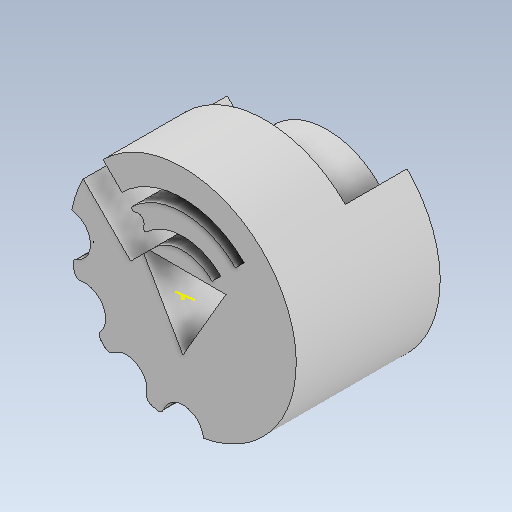
# Autodesk Inventor part: HandleGear
Saved by Autodesk Inventor 2021 (Build 250183000, 183)
## iProperties
Created: 2021-03-14
Part Number: HandleGear
Material: Generic
Document SubType Name: Modeling
Designer: ben
Density: 1 g/cm^3
Appearance: Default
Mass: 73.1754 g
Surface Area: 125.549 cm^2
Volume: 73.1754 cm^3
Author: ben
Autodesk Inventor part; units mm, degrees
ref_plane "YZ Plane" through (0, 0, 0) normal (1, 0, 0) x (0, 1, 0)
ref_plane "XZ Plane" through (0, 0, 0) normal (0, 1, 0) x (-1, 0, 0)
ref_plane "XY Plane" through (0, 0, 0) normal (0, 0, 1) x (1, 0, 0)
sketch "Sketch1" plane through (0, 0, 0) normal (0, 0, 1) x (1, 0, 0)
  line L0 (5.1877, -3.0147) -> (-0.0339, -12) projected
  line L1 (-0.0339, -12) -> (-5.2046, -2.9853) projected
  line L2 (-10.3753, 6.0293) -> (0.0169, 6) projected
  circle A0 centre (0, 0) radius 27.5 projected
  circle A1 centre (0, 0) radius 22.5
  line L3 (0, 27.5) -> (0, 14.4902)
  line L4 (0, 0) -> (27.5, 0) construction
  line L5 (0, 0) -> (27.5, 0) construction
  circle A2 centre (-27.5, 0) radius 5
  circle A3 centre (-23.8157, -13.75) radius 5
  circle A4 centre (-13.75, -23.8157) radius 5
  circle A5 centre (0, -27.5) radius 5
  line L6 (-5.2046, -2.9853) -> (-10.3753, 6.0293) projected
  line L7 (0.0169, 6) -> (10.4092, 5.9706) projected
  line L8 (10.4092, 5.9706) -> (5.1877, -3.0147) projected
  arc A6 (7.0711, 7.0711) -> (-7.0711, 7.0711) centre (0, 0) ccw
  line L9 (0, 0) -> (-7.0711, 7.0711) construction
  line L10 (0, 0) -> (10, 0) construction
  line L11 (0, 0) -> (7.0711, 7.0711) construction
  arc A7 (9.1924, 9.1924) -> (-9.1924, 9.1924) centre (0, 0) ccw
  line L12 (0, 0) -> (-9.1924, 9.1924) construction
  line L13 (0, 0) -> (13, 0) construction
  line L14 (0, 0) -> (9.1924, 9.1924) construction
  arc A8 (12.7279, 12.7279) -> (-12.7279, 12.7279) centre (0, 0) ccw
  line L15 (0, 0) -> (-12.7279, 12.7279) construction
  line L16 (0, 0) -> (18, 0) construction
  line L17 (0, 0) -> (12.7279, 12.7279) construction
  arc A9 (14.8492, 14.8492) -> (-14.8492, 14.8492) centre (0, 0) ccw
  line L18 (0, 0) -> (19, 0) construction
  line L19 (0, 0) -> (14.8492, 14.8492) construction
  line L20 (-7.0711, 7.0711) -> (-9.1924, 9.1924)
  line L21 (-9.1924, 9.1924) -> (-12.7279, 12.7279)
  line L22 (-14.8492, 14.8492) -> (-12.7279, 12.7279)
  line L23 (7.0711, 7.0711) -> (9.1924, 9.1924)
  line L24 (9.1924, 9.1924) -> (12.7279, 12.7279)
  line L25 (14.8492, 14.8492) -> (12.7279, 12.7279)
  line L26 (-7.0711, 7.0711) -> (-9.1924, 9.1924)
  line L27 (-9.1924, 9.1924) -> (-12.7279, 12.7279)
  line L28 (-14.8492, 14.8492) -> (-12.7279, 12.7279)
  line L29 (-7.0711, 7.0711) -> (-19.4454, 19.4454)
  line L30 (-19.4454, 19.4454) -> (-25.1023, 13.7886)
  line L31 (-25.1023, 13.7886) -> (-12.7279, 1.4142)
  line L32 (-12.7279, 1.4142) -> (-7.0711, 7.0711)
  arc A10 (16.9706, 16.9706) -> (-16.9706, 16.9706) centre (0, 0) ccw
  line L33 (-14.8492, 14.8492) -> (-16.9706, 16.9706)
  line L34 (14.8492, 14.8492) -> (16.9706, 16.9706)
  arc A11 (-9.8995, 9.8995) -> (-12.0208, 12.0208) centre (-10.9602, 10.9602) ccw
  point P0 (0, 0)
  point P1 (-27.0822, 4.7753)
  point P2 (4.7753, -27.0822)
  point P3 (-4.9793, -27.0455)
  point P4 (4.9793, -27.0455)
  point P5 (-27.0455, 4.9793)
  point P6 (-27.0455, -4.9793)
  point P7 (-25.9117, -9.2105)
  point P8 (-20.9324, -17.8349)
  point P9 (-17.8349, -20.9324)
  point P10 (-9.2105, -25.9117)
  point P11 (0, -22.5)
  point P12 (-11.25, -19.4856)
  point P13 (-19.4856, -11.25)
  point P14 (-22.5, 0)
  point P15 (-27.0455, 4.9793)
  point P16 (4.9793, -27.0455)
  point P17 (-24.2613, 12.9476)
  dimension "d9" = 10
  dimension "d0" = 5
  dimension "d12" = 90
  dimension "d70" = 10
  dimension "d71" = 135
  dimension "d72" = 90
  dimension "d73" = 13
  dimension "d74" = 135
  dimension "d75" = 90
  dimension "d76" = 18
  dimension "d77" = 135
  dimension "d78" = 90
  dimension "d79" = 21
  dimension "d88" = 8
  dimension "d93" = 24
  dimension "d94" = 3
  constraints: 58 end point, 14 point on circle, 9 centre point, 6 horizontal, 5 coincident, 5 point on line, 3 equal length, 2 parallel, 2 vertical, 1 perpendicular, 21 other
  measures "d70" radius of A6
  measures "d71" angle of L10 L9
  measures "d72" angle of L11 L9
  measures "d73" radius of A7
  measures "d74" angle of L13 L12
  measures "d75" angle of L14 L12
  measures "d76" radius of A8
  measures "d77" angle of L16 L15
  measures "d78" angle of L17 L15
  measures "d79" radius of A9
  measures "d88" distance of L30.end L29.end
  measures "d93" radius of A10
  measures "d94" diameter of A11
extrude "Extrusion6" add sketch "Sketch1" along normal blind 35 contours L8 L7 L2 L32 A6 L23 L24 L25 L34 A1 L31 L6 L1 L0 | A1 A2 A0 L31 | L21 A11 A8 L24 A7 | L29 A10 L3 A1 | A1 L3 A9 L29 | A1 A3 A0 A2 | L3 A10 L34 A1 | A1 L34 A9 L3 | L29 A0 L3 A10 | A1 A4 A0 A3 | L34 A10 L3 A0 A5 A1 | A1 A5 A0 A4
sketch "Sketch7" plane through (0, 0, 0) normal (0, 0, -1) x (-1, 0, 0)
  line L0 (8.6461, 5.0244) -> (4.3372, -2.4878)
  arc A0 (-4.323, -2.5122) -> (4.3372, -2.4878) centre (0, 0) ccw
  line L1 (0.0282, -10) -> (-4.323, -2.5122)
  line L2 (4.3372, -2.4878) -> (0.0282, -10)
  arc A1 (4.3372, -2.4878) -> (-0.0141, 5) centre (0, 0) ccw
  line L3 (-0.0141, 5) -> (8.6461, 5.0244)
  arc A2 (-0.0141, 5) -> (-4.323, -2.5122) centre (0, 0) ccw
  line L4 (-4.323, -2.5122) -> (-8.6743, 4.9755)
  line L5 (-8.6743, 4.9755) -> (-0.0141, 5)
  circle A3 centre (0, 0) radius 27.5
  spline S0 degree 2 poles (19.7349, 0.4642) (19.3981, 0.44) (19.187, 0.6034) knots 0 0 0 1 1 1
  spline S1 degree 2 poles (19.187, 0.6034) (18.9616, 0.7727) (18.9378, 1.1048) knots 0 0 0 1 1 1
  line L6 (18.9378, 1.1048) -> (18.8689, 2.0666)
  line L7 (18.8689, 2.0666) -> (17.5058, 1.9689)
  spline S2 degree 2 poles (17.5058, 1.9689) (17.3651, 1.9588) (17.3555, 2.0926) knots 0 0 0 1 1 1
  spline S3 degree 2 poles (17.3555, 2.0926) (17.3457, 2.2287) (17.4864, 2.2388) knots 0 0 0 1 1 1
  line L8 (17.4864, 2.2388) -> (20.3787, 2.4461)
  line L9 (20.3787, 2.4461) -> (20.4617, 1.2882)
  spline S4 degree 2 poles (20.4617, 1.2882) (20.4895, 0.9008) (20.2823, 0.6865) knots 0 0 0 1 1 1
  spline S5 degree 2 poles (20.2823, 0.6865) (20.0924, 0.4898) (19.7349, 0.4642) knots 0 0 0 1 1 1
  spline S6 degree 2 poles (19.7155, 0.734) (20.2229, 0.7704) (20.1872, 1.2686) knots 0 0 0 1 1 1
  line L10 (20.1872, 1.2686) -> (20.1236, 2.1566)
  line L11 (20.1236, 2.1566) -> (19.148, 2.0866)
  line L12 (19.148, 2.0866) -> (19.2169, 1.1248)
  spline S7 degree 2 poles (19.2169, 1.1248) (19.2314, 0.9219) (19.5033, 0.7188) (19.7155, 0.734) knots 0 0 0 1 2 2 2
  spline S8 degree 2 poles (18.4359, -2.1408) (17.8385, -2.0989) (17.5674, -1.6672) knots 0 0 0 1 1 1
  spline S9 degree 2 poles (17.5674, -1.6672) (17.3177, -1.2626) (17.4853, -0.8223) knots 0 0 0 1 1 1
  spline S10 degree 2 poles (17.4853, -0.8223) (17.664, -0.3574) (18.1971, -0.2255) knots 0 0 0 1 1 1
  spline S11 degree 2 poles (18.1971, -0.2255) (18.2254, -0.2183) (18.2462, -0.2197) knots 0 0 0 1 1 1
  spline S12 degree 2 poles (18.2462, -0.2197) (18.3754, -0.2288) (18.3658, -0.3649) knots 0 0 0 1 1 1
  spline S13 degree 2 poles (18.3658, -0.3649) (18.3592, -0.4594) (18.2625, -0.4828) knots 0 0 0 1 1 1
  spline S14 degree 2 poles (18.2625, -0.4828) (18.0102, -0.5439) (17.8653, -0.7261) knots 0 0 0 1 1 1
  spline S15 degree 2 poles (17.8653, -0.7261) (17.7287, -0.8881) (17.7135, -1.1049) knots 0 0 0 1 1 1
  spline S16 degree 2 poles (17.7135, -1.1049) (17.6935, -1.3909) (17.8822, -1.6082) knots 0 0 0 1 1 1
  spline S17 degree 2 poles (17.8822, -1.6082) (18.0878, -1.8498) (18.4545, -1.8755) knots 0 0 0 1 1 1
  spline S18 degree 2 poles (18.4545, -1.8755) (18.8375, -1.9024) (19.0519, -1.6879) knots 0 0 0 1 1 1
  spline S19 degree 2 poles (19.0519, -1.6879) (19.2113, -1.5299) (19.275, -1.2493) knots 0 0 0 1 1 1
  spline S20 degree 2 poles (19.275, -1.2493) (19.2948, -1.1) (19.3452, -0.8114) (19.4236, -0.8169) knots 0 0 0 1 2 2 2
  spline S21 degree 2 poles (19.4236, -0.8169) (19.4951, -0.8219) (19.5573, -0.8935) knots 0 0 0 1 1 1
  line L13 (19.5573, -0.8935) -> (20.1606, -1.578)
  line L14 (20.1606, -1.578) -> (20.2268, -0.6345)
  spline S22 degree 2 poles (20.2268, -0.6345) (20.2365, -0.4961) (20.375, -0.5058) knots 0 0 0 1 1 1
  spline S23 degree 2 poles (20.375, -0.5058) (20.511, -0.5154) (20.5013, -0.6538) knots 0 0 0 1 1 1
  line L15 (20.5013, -0.6538) -> (20.4109, -2.0081)
  spline S24 degree 2 poles (20.4109, -2.0081) (20.4035, -2.1142) (20.3343, -2.1094) knots 0 0 0 1 1 1
  spline S25 degree 2 poles (20.3343, -2.1094) (20.2766, -2.1053) (20.1542, -1.9669) knots 0 0 0 1 1 1
  line L16 (20.1542, -1.9669) -> (19.5542, -1.3013)
  spline S26 degree 2 poles (19.5542, -1.3013) (19.3678, -2.2062) (18.4359, -2.1408) knots 0 0 0 1 1 1
  spline S27 degree 2 poles (17.298, -9.511) (16.9947, -9.3627) (16.8943, -9.1154) knots 0 0 0 1 1 1
  spline S28 degree 2 poles (16.8943, -9.1154) (16.7844, -8.8558) (16.9306, -8.5567) knots 0 0 0 1 1 1
  line L17 (16.9306, -8.5567) -> (17.3541, -7.6904)
  line L18 (17.3541, -7.6904) -> (16.1263, -7.0902)
  spline S29 degree 2 poles (16.1263, -7.0902) (15.9996, -7.0283) (16.0585, -6.9078) knots 0 0 0 1 1 1
  spline S30 degree 2 poles (16.0585, -6.9078) (16.1184, -6.7852) (16.2451, -6.8471) knots 0 0 0 1 1 1
  line L19 (16.2451, -6.8471) -> (18.8502, -8.1206)
  line L20 (18.8502, -8.1206) -> (18.3404, -9.1635)
  spline S31 degree 2 poles (18.3404, -9.1635) (18.1698, -9.5125) (17.8831, -9.5936) knots 0 0 0 1 1 1
  spline S32 degree 2 poles (17.8831, -9.5936) (17.62, -9.6684) (17.298, -9.511) knots 0 0 0 1 1 1
  spline S33 degree 2 poles (17.4168, -9.2679) (17.8739, -9.4913) (18.0932, -9.0426) knots 0 0 0 1 1 1
  line L21 (18.0932, -9.0426) -> (18.4842, -8.2428)
  line L22 (18.4842, -8.2428) -> (17.6054, -7.8132)
  line L23 (17.6054, -7.8132) -> (17.182, -8.6795)
  spline S34 degree 2 poles (17.182, -8.6795) (17.0926, -8.8623) (17.2257, -9.1745) (17.4168, -9.2679) knots 0 0 0 1 2 2 2
  line L24 (14.13, -10.3544) -> (15.073, -8.9571)
  spline S35 degree 2 poles (15.073, -8.9571) (15.2622, -9.1769) (15.447, -9.3909) knots 0 0 0 1 1 1
  spline S36 degree 2 poles (15.447, -9.3909) (15.6884, -9.6988) (15.7955, -10.0278) knots 0 0 0 1 1 1
  spline S37 degree 2 poles (15.7955, -10.0278) (15.9386, -10.4647) (15.8925, -11.0333) knots 0 0 0 1 1 1
  spline S38 degree 2 poles (15.8925, -11.0333) (15.8623, -11.3756) (16.1057, -11.5399) knots 0 0 0 1 1 1
  spline S39 degree 2 poles (16.1057, -11.5399) (16.2552, -11.6408) (16.435, -11.6059) knots 0 0 0 1 1 1
  spline S40 degree 2 poles (16.435, -11.6059) (16.6232, -11.5627) (16.7512, -11.3729) knots 0 0 0 1 1 1
  spline S41 degree 2 poles (16.7512, -11.3729) (16.8935, -11.1621) (16.9111, -11.0038) knots 0 0 0 1 1 1
  spline S42 degree 2 poles (16.9111, -11.0038) (16.9243, -10.8147) (16.7812, -10.6009) knots 0 0 0 1 1 1
  spline S43 degree 2 poles (16.7812, -10.6009) (16.7316, -10.5256) (16.7769, -10.4585) knots 0 0 0 1 1 1
  spline S44 degree 2 poles (16.7769, -10.4585) (16.8532, -10.3454) (16.9644, -10.4205) knots 0 0 0 1 1 1
  spline S45 degree 2 poles (16.9644, -10.4205) (16.9855, -10.4347) (17.0026, -10.463) knots 0 0 0 1 1 1
  spline S46 degree 2 poles (17.0026, -10.463) (17.3505, -10.9851) (16.9935, -11.5141) knots 0 0 0 1 1 1
  spline S47 degree 2 poles (16.9935, -11.5141) (16.784, -11.8246) (16.4809, -11.8935) knots 0 0 0 1 1 1
  spline S48 degree 2 poles (16.4809, -11.8935) (16.2034, -11.9573) (15.9619, -11.7943) knots 0 0 0 1 1 1
  spline S49 degree 2 poles (15.9619, -11.7943) (15.5843, -11.5395) (15.6239, -11.0055) knots 0 0 0 1 1 1
  spline S50 degree 2 poles (15.6239, -11.0055) (15.671, -10.3817) (15.4785, -9.9561) knots 0 0 0 1 1 1
  spline S51 degree 2 poles (15.4785, -9.9561) (15.3796, -9.7471) (15.0954, -9.4158) knots 0 0 0 1 1 1
  line L25 (15.0954, -9.4158) -> (14.3581, -10.5084)
  spline S52 degree 2 poles (14.3581, -10.5084) (14.2805, -10.6234) (14.1674, -10.5471) knots 0 0 0 1 1 1
  spline S53 degree 2 poles (14.1674, -10.5471) (14.0524, -10.4694) (14.13, -10.3544) knots 0 0 0 1 1 1
  spline S54 degree 2 poles (9.6963, -17.1948) (9.5165, -16.9091) (9.5614, -16.6459) knots 0 0 0 1 1 1
  spline S55 degree 2 poles (9.5614, -16.6459) (9.6047, -16.3674) (9.8865, -16.1901) knots 0 0 0 1 1 1
  line L26 (9.8865, -16.1901) -> (10.7027, -15.6766)
  line L27 (10.7027, -15.6766) -> (9.9751, -14.5199)
  spline S56 degree 2 poles (9.9751, -14.5199) (9.9, -14.4005) (10.0135, -14.3291) knots 0 0 0 1 1 1
  spline S57 degree 2 poles (10.0135, -14.3291) (10.129, -14.2564) (10.2041, -14.3758) knots 0 0 0 1 1 1
  line L28 (10.2041, -14.3758) -> (11.748, -16.8303)
  line L29 (11.748, -16.8303) -> (10.7655, -17.4484)
  spline S58 degree 2 poles (10.7655, -17.4484) (10.4366, -17.6552) (10.1501, -17.5732) knots 0 0 0 1 1 1
  spline S59 degree 2 poles (10.1501, -17.5732) (9.8871, -17.4982) (9.6963, -17.1948) knots 0 0 0 1 1 1
  spline S60 degree 2 poles (9.9253, -17.0508) (10.1962, -17.4814) (10.619, -17.2154) knots 0 0 0 1 1 1
  line L30 (10.619, -17.2154) -> (11.3725, -16.7414)
  line L31 (11.3725, -16.7414) -> (10.8517, -15.9135)
  line L32 (10.8517, -15.9135) -> (10.0355, -16.4269)
  spline S61 degree 2 poles (10.0355, -16.4269) (9.8633, -16.5353) (9.812, -16.8707) (9.9253, -17.0508) knots 0 0 0 1 2 2 2
  spline S62 degree 2 poles (7.6271, -15.8637) (7.5674, -15.7411) (7.6879, -15.6823) knots 0 0 0 1 1 1
  spline S63 degree 2 poles (7.6879, -15.6823) (7.8106, -15.6225) (7.8703, -15.7452) knots 0 0 0 1 1 1
  line L33 (7.8703, -15.7452) -> (9.0811, -18.2291)
  spline S64 degree 2 poles (9.0811, -18.2291) (9.1409, -18.3517) (9.0182, -18.4115) knots 0 0 0 1 1 1
  spline S65 degree 2 poles (9.0182, -18.4115) (8.8977, -18.4702) (8.8379, -18.3476) knots 0 0 0 1 1 1
  line L34 (8.8379, -18.3476) -> (7.6271, -15.8637)
  spline S66 degree 2 poles (1.6734, -18.9273) (1.5826, -18.3143) (1.8076, -17.8439) knots 0 0 0 1 1 1
  spline S67 degree 2 poles (1.8076, -17.8439) (2.0538, -17.3282) (2.5662, -17.2524) knots 0 0 0 1 1 1
  spline S68 degree 2 poles (2.5662, -17.2524) (3.074, -17.1772) (3.4682, -17.5981) knots 0 0 0 1 1 1
  spline S69 degree 2 poles (3.4682, -17.5981) (3.8348, -17.9903) (3.9242, -18.5942) knots 0 0 0 1 1 1
  spline S70 degree 2 poles (3.9242, -18.5942) (4.0143, -19.2026) (3.797, -19.693) knots 0 0 0 1 1 1
  spline S71 degree 2 poles (3.797, -19.693) (3.5577, -20.2239) (3.0659, -20.2967) knots 0 0 0 1 1 1
  spline S72 degree 2 poles (3.0659, -20.2967) (2.5397, -20.3746) (2.1363, -19.9387) knots 0 0 0 1 1 1
  spline S73 degree 2 poles (2.1363, -19.9387) (1.7634, -19.5358) (1.6734, -18.9273) knots 0 0 0 1 1 1
  spline S74 degree 2 poles (1.941, -18.8877) (2.0162, -19.3955) (2.2928, -19.7169) knots 0 0 0 1 1 1
  spline S75 degree 2 poles (2.2928, -19.7169) (2.6017, -20.0826) (3.0249, -20.0199) knots 0 0 0 1 1 1
  spline S76 degree 2 poles (3.0249, -20.0199) (3.4183, -19.9617) (3.5829, -19.5259) knots 0 0 0 1 1 1
  spline S77 degree 2 poles (3.5829, -19.5259) (3.7278, -19.1469) (3.652, -18.6345) knots 0 0 0 1 1 1
  spline S78 degree 2 poles (3.652, -18.6345) (3.5775, -18.1312) (3.3107, -17.8131) knots 0 0 0 1 1 1
  spline S79 degree 2 poles (3.3107, -17.8131) (3.0137, -17.4643) (2.6065, -17.5246) knots 0 0 0 1 1 1
  spline S80 degree 2 poles (2.6065, -17.5246) (2.1948, -17.5855) (2.0206, -18.004) knots 0 0 0 1 1 1
  spline S81 degree 2 poles (2.0206, -18.004) (1.8658, -18.3799) (1.941, -18.8877) knots 0 0 0 1 1 1
  line L35 (-0.961, -20.2153) -> (0.6229, -20.2266)
  line L36 (0.6229, -20.2266) -> (0.6296, -19.2925)
  line L37 (0.6296, -19.2925) -> (-0.5959, -19.2837)
  spline S82 degree 2 poles (-0.5959, -19.2837) (-0.737, -19.2827) (-0.736, -19.1462) knots 0 0 0 1 1 1
  spline S83 degree 2 poles (-0.736, -19.1462) (-0.735, -19.0075) (-0.5939, -19.0085) knots 0 0 0 1 1 1
  line L38 (-0.5939, -19.0085) -> (0.6316, -19.0173)
  line L39 (0.6316, -19.0173) -> (0.6416, -17.6207)
  spline S84 degree 2 poles (0.6416, -17.6207) (0.6426, -17.4796) (0.7767, -17.4806) knots 0 0 0 1 1 1
  spline S85 degree 2 poles (0.7767, -17.4806) (0.9131, -17.4815) (0.9121, -17.6226) knots 0 0 0 1 1 1
  line L40 (0.9121, -17.6226) -> (0.8915, -20.5037)
  line L41 (0.8915, -20.5037) -> (-0.963, -20.4904)
  spline S86 degree 2 poles (-0.963, -20.4904) (-1.0994, -20.4895) (-1.0984, -20.353) knots 0 0 0 1 1 1
  spline S87 degree 2 poles (-1.0984, -20.353) (-1.0974, -20.2143) (-0.961, -20.2153) knots 0 0 0 1 1 1
  line L42 (-3.9103, -19.8568) -> (-2.3451, -20.0999)
  line L43 (-2.3451, -20.0999) -> (-2.2017, -19.1768)
  line L44 (-2.2017, -19.1768) -> (-3.4127, -18.9887)
  spline S88 degree 2 poles (-3.4127, -18.9887) (-3.5521, -18.967) (-3.5312, -18.8322) knots 0 0 0 1 1 1
  spline S89 degree 2 poles (-3.5312, -18.8322) (-3.5099, -18.6951) (-3.3705, -18.7167) knots 0 0 0 1 1 1
  line L45 (-3.3705, -18.7167) -> (-2.1595, -18.9048)
  line L46 (-2.1595, -18.9048) -> (-1.9451, -17.5247)
  spline S90 degree 2 poles (-1.9451, -17.5247) (-1.9234, -17.3853) (-1.7909, -17.4059) knots 0 0 0 1 1 1
  spline S91 degree 2 poles (-1.7909, -17.4059) (-1.6561, -17.4269) (-1.6777, -17.5662) knots 0 0 0 1 1 1
  line L47 (-1.6777, -17.5662) -> (-2.12, -20.4133)
  line L48 (-2.12, -20.4133) -> (-3.9525, -20.1287)
  spline S92 degree 2 poles (-3.9525, -20.1287) (-4.0873, -20.1077) (-4.0664, -19.9729) knots 0 0 0 1 1 1
  spline S93 degree 2 poles (-4.0664, -19.9729) (-4.0451, -19.8358) (-3.9103, -19.8568) knots 0 0 0 1 1 1
  point P0 (0, 0)
  constraints: 12 end point, 6 point on circle, 4 centre point, 24 other
emboss "Emboss1" sketch "Sketch7" operation cut depth 1 direction (0, 0, 1) contours S0 S1 L6 L7 S2 S3 L8 L9 S4 S5 | S8 S9 S10 S11 S12 S13 S14 S15 S16 S17 S18 S19 S20 S21 L13 L14 S22 S23 L15 S24 S25 L16 S26 | S27 S28 L17 L18 S29 S30 L19 L20 S31 S32 | L24 S35 S36 S37 S38 S39 S40 S41 S42 S43 S44 S45 S46 S47 S48 S49 S50 S51 L25 S52 S53 | S54 S55 L26 L27 S56 S57 L28 L29 S58 S59 | S62 S63 L33 S64 S65 L34 | S66 S67 S68 S69 S70 S71 S72 S73 | L35 L36 L37 S82 S83 L38 L39 S84 S85 L40 L41 S86 S87 | L42 L43 L44 S88 S89 L45 L46 S90 S91 L47 L48 S92 S93
fillet "Fillet7" radius 1.5 6 edges at (-27.0455, -4.9793, 17.5) (-25.9117, -9.2105, 17.5) (-20.9324, -17.8349, 17.5) (-17.8349, -20.9324, 17.5) (-9.2105, -25.9117, 17.5) (-4.9793, -27.0455, 17.5)
fillet "Fillet8" radius 0.5 4 edges at (-12.7279, 12.7279, 17.5) (-9.1924, 9.1924, 17.5) (-12.0208, 12.0208, 17.5) (-9.8995, 9.8995, 17.5)
sketch "Sketch8" plane through (0, 0, 0) normal (0, 0, -1) x (-1, 0, 0)
  line L0 (-1.9451, -17.5247) -> (-2.1595, -18.9048) projected
  line L1 (-2.1595, -18.9048) -> (-3.3705, -18.7167) projected
  line L2 (-3.4127, -18.9887) -> (-2.2017, -19.1768) projected
  line L3 (-2.2017, -19.1768) -> (-2.3451, -20.0999) projected
  line L4 (-2.3451, -20.0999) -> (-3.9103, -19.8568) projected
  line L5 (-3.9525, -20.1287) -> (-2.12, -20.4133) projected
  line L6 (-2.12, -20.4133) -> (-1.6777, -17.5662) projected
  line L7 (19.2169, 1.1248) -> (19.148, 2.0866) projected
  line L8 (19.148, 2.0866) -> (20.1236, 2.1566) projected
  line L9 (20.1236, 2.1566) -> (20.1872, 1.2686) projected
  line L10 (17.5058, 1.9689) -> (18.8689, 2.0666) projected
  line L11 (18.8689, 2.0666) -> (18.9378, 1.1048) projected
  line L12 (20.4617, 1.2882) -> (20.3787, 2.4461) projected
  line L13 (20.3787, 2.4461) -> (17.4864, 2.2388) projected
  line L14 (18.3404, -9.1635) -> (18.8502, -8.1206) projected
  line L15 (18.8502, -8.1206) -> (16.2451, -6.8471) projected
  line L16 (16.1263, -7.0902) -> (17.3541, -7.6904) projected
  line L17 (17.3541, -7.6904) -> (16.9306, -8.5567) projected
  line L18 (17.182, -8.6795) -> (17.6054, -7.8132) projected
  line L19 (17.6054, -7.8132) -> (18.4842, -8.2428) projected
  line L20 (18.4842, -8.2428) -> (18.0932, -9.0426) projected
  line L21 (19.5542, -1.3013) -> (20.1542, -1.9669) projected
  line L22 (20.4109, -2.0081) -> (20.5013, -0.6538) projected
  line L23 (20.2268, -0.6345) -> (20.1606, -1.578) projected
  line L24 (20.1606, -1.578) -> (19.5573, -0.8935) projected
  line L25 (15.073, -8.9571) -> (14.13, -10.3544) projected
  line L26 (14.3581, -10.5084) -> (15.0954, -9.4158) projected
  line L27 (10.0355, -16.4269) -> (10.8517, -15.9135) projected
  line L28 (10.8517, -15.9135) -> (11.3725, -16.7414) projected
  line L29 (11.3725, -16.7414) -> (10.619, -17.2154) projected
  line L30 (9.9751, -14.5199) -> (10.7027, -15.6766) projected
  line L31 (10.7027, -15.6766) -> (9.8865, -16.1901) projected
  line L32 (10.7655, -17.4484) -> (11.748, -16.8303) projected
  line L33 (11.748, -16.8303) -> (10.2041, -14.3758) projected
  line L34 (9.0811, -18.2291) -> (7.8703, -15.7452) projected
  line L35 (7.6271, -15.8637) -> (8.8379, -18.3476) projected
  line L36 (0.6229, -20.2266) -> (-0.961, -20.2153) projected
  line L37 (-0.963, -20.4904) -> (0.8915, -20.5037) projected
  line L38 (0.8915, -20.5037) -> (0.9121, -17.6226) projected
  line L39 (0.6416, -17.6207) -> (0.6316, -19.0173) projected
  line L40 (0.6316, -19.0173) -> (-0.5939, -19.0085) projected
  line L41 (-0.5959, -19.2837) -> (0.6296, -19.2925) projected
  line L42 (0.6296, -19.2925) -> (0.6229, -20.2266) projected
  line L43 (8.1192, 6.023) -> (-10.4092, 5.9706) projected
  line L44 (-10.4092, 5.9706) -> (0.0339, -12) projected
  line L45 (0.0339, -12) -> (9.5506, 4.5915) projected
  line L46 (9.5506, 4.5915) -> (12.7279, 1.4142) projected
  line L47 (12.7279, 1.4142) -> (24.2613, 12.9476) projected
  arc A0 (27.0455, 4.9793) -> (24.2613, 12.9476) centre (0, 0) ccw projected
  arc A1 (27.0455, 4.9793) -> (25.7867, -4.6973) centre (27.5, 0) ccw projected
  arc A2 (26.7308, -6.4588) -> (25.7867, -4.6973) centre (25.2727, -6.1065) ccw projected
  arc A3 (26.3789, -7.7719) -> (26.7308, -6.4588) centre (0, 0) ccw projected
  arc A4 (24.6806, -8.8254) -> (26.3789, -7.7719) centre (24.9401, -7.348) ccw projected
  arc A5 (24.6806, -8.8254) -> (19.9833, -16.9613) centre (23.8157, -13.75) ccw projected
  arc A6 (19.9201, -18.9589) -> (19.9833, -16.9613) centre (18.8336, -17.9247) ccw projected
  arc A7 (18.9589, -19.9201) -> (19.9201, -18.9589) centre (0, 0) ccw projected
  arc A8 (16.9613, -19.9833) -> (18.9589, -19.9201) centre (17.9247, -18.8336) ccw projected
  arc A9 (16.9613, -19.9833) -> (8.8254, -24.6806) centre (13.75, -23.8157) ccw projected
  arc A10 (7.7719, -26.3789) -> (8.8254, -24.6806) centre (7.348, -24.9401) ccw projected
  arc A11 (6.4588, -26.7308) -> (7.7719, -26.3789) centre (0, 0) ccw projected
  arc A12 (4.6973, -25.7867) -> (6.4588, -26.7308) centre (6.1065, -25.2727) ccw projected
  arc A13 (4.6973, -25.7867) -> (-4.9793, -27.0455) centre (0, -27.5) ccw projected
  arc A14 (19.4454, 19.4454) -> (-4.9793, -27.0455) centre (0, 0) ccw projected
  line L48 (19.4454, 19.4454) -> (14.8492, 14.8492) projected
  arc A15 (14.8492, 14.8492) -> (-14.8492, 14.8492) centre (0, 0) ccw projected
  line L49 (-14.8492, 14.8492) -> (-12.7279, 12.7279) projected
  arc A16 (12.3591, 13.0864) -> (-12.7279, 12.7279) centre (0, 0) ccw projected
  line L50 (9.5908, 9.5908) -> (9.5394, 9.5394) projected
  arc A17 (8.8456, 9.5265) -> (9.5394, 9.5394) centre (9.1858, 9.8929) ccw projected
  arc A18 (8.8456, 9.5265) -> (-9.1924, 9.1924) centre (0, 0) ccw projected
  line L51 (-9.1924, 9.1924) -> (-7.0711, 7.0711) projected
  arc A19 (7.0711, 7.0711) -> (-7.0711, 7.0711) centre (0, 0) ccw projected
  arc A20 (14.8492, 14.8492) -> (-14.8492, 14.8492) centre (0, 0) ccw projected
  arc A21 (14.8492, 14.8492) -> (-14.8492, 14.8492) centre (0, 0) ccw
  line L52 (19.4454, 19.4454) -> (14.8492, 14.8492) projected
  arc A22 (19.4454, 19.4454) -> (-19.4454, 19.4454) centre (0, 0) ccw
  line L53 (-14.8492, 14.8492) -> (-19.4454, 19.4454)
  arc A23 (12.3693, 12.3693) -> (12.3591, 13.0864) centre (12.0158, 12.7229) ccw projected
  line L54 (12.3693, 12.3693) -> (12.3295, 12.3295) projected
  arc A24 (11.722, 12.2523) -> (12.3295, 12.3295) centre (11.9759, 12.683) ccw projected
  arc A25 (11.722, 12.2523) -> (9.668, 10.1983) centre (10.9602, 10.9602) ccw projected
  arc A26 (9.5908, 9.5908) -> (9.668, 10.1983) centre (9.2373, 9.9444) ccw projected
  line L55 (7.0711, 7.0711) -> (8.1192, 6.023) projected
  point P0 (0, 0)
  point P1 (-19.4454, 19.4454)
  constraints: 4 point on circle, 2 centre point, 2 coincident, 2 end point, 94 other
extrude "Extrusion7" cut sketch "Sketch8" against normal blind 15 contours L53 A14 L48 A15
sketch "Sketch10" plane through (0, 0, 35) normal (0, 0, 1) x (1, 0, 0)
  line L0 (-1.9897, 0.4439) -> (2.6094, 1.062) projected
  point P0 (0, 0)
body "Solid3"
